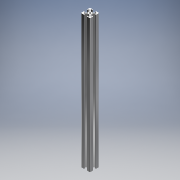
# Autodesk Inventor part: 400mm
Saved by Autodesk Inventor 2017 (Build 210142000, 142)
## iProperties
Part Number: 400mm
Material: Aluminium 6061
Document SubType Name: Modeling
Designer: Till
Density: 2.7 g/cm^3
Appearance: Aluminium - flach
Author: Till
Autodesk Inventor part; units mm, degrees
ref_plane "YZ Plane" through (0, 0, 0) normal (1, 0, 0) x (0, 1, 0)
ref_plane "XZ Plane" through (0, 0, 0) normal (0, 1, 0) x (-1, 0, 0)
ref_plane "XY Plane" through (0, 0, 0) normal (0, 0, 1) x (1, 0, 0)
sketch "Skizze1" plane through (0, 0, 0) normal (0, 0, 1) x (1, 0, 0)
  circle A0 centre (0, 0) radius 2.15
  line L0 (-3.5, -9.5) -> (-3.5, -10)
  line L1 (-3, -9.5) -> (-3.5, -9.5)
  line L2 (-3, -8.3) -> (-3, -9.5)
  line L3 (-5.2994, -8.3) -> (-3, -8.3)
  arc A1 (-5.7944, -7.105) -> (-5.2994, -8.3) centre (-5.2994, -7.6) ccw
  line L4 (-2.1755, -3.4861) -> (-5.7944, -7.105)
  arc A2 (-1.6076, -3.388) -> (-2.1755, -3.4861) centre (-1.8219, -3.8397) ccw
  arc A3 (-1.6076, -3.388) -> (-0.3, -3.738) centre (0, 0) ccw
  line L5 (0, -3.45) -> (-0.3, -3.738)
  line L6 (0.3, -3.738) -> (0, -3.45)
  arc A4 (0.3, -3.738) -> (1.6076, -3.388) centre (0, 0) ccw
  arc A5 (2.1755, -3.4861) -> (1.6076, -3.388) centre (1.8219, -3.8397) ccw
  line L7 (5.7944, -7.105) -> (2.1755, -3.4861)
  arc A6 (5.2994, -8.3) -> (5.7944, -7.105) centre (5.2994, -7.6) ccw
  line L8 (3, -8.3) -> (5.2994, -8.3)
  line L9 (3, -9.5) -> (3, -8.3)
  line L10 (3.5, -9.5) -> (3, -9.5)
  line L11 (3.5, -10) -> (3.5, -9.5)
  line L12 (8.5, -10) -> (3.5, -10)
  arc A7 (8.5, -10) -> (10, -8.5) centre (8.5, -8.5) ccw
  line L13 (10, -3.5) -> (10, -8.5)
  line L14 (9.5, -3.5) -> (10, -3.5)
  line L15 (9.5, -3) -> (9.5, -3.5)
  line L16 (8.3, -3) -> (9.5, -3)
  line L17 (8.3, -5.2994) -> (8.3, -3)
  arc A8 (7.105, -5.7944) -> (8.3, -5.2994) centre (7.6, -5.2994) ccw
  line L18 (3.4861, -2.1755) -> (7.105, -5.7944)
  arc A9 (3.388, -1.6076) -> (3.4861, -2.1755) centre (3.8397, -1.8219) ccw
  arc A10 (3.388, -1.6076) -> (3.738, -0.3) centre (0, 0) ccw
  line L19 (3.45, 0) -> (3.738, -0.3)
  line L20 (3.738, 0.3) -> (3.45, 0)
  arc A11 (3.738, 0.3) -> (3.388, 1.6076) centre (0, 0) ccw
  arc A12 (3.4861, 2.1755) -> (3.388, 1.6076) centre (3.8397, 1.8219) ccw
  line L21 (7.105, 5.7944) -> (3.4861, 2.1755)
  arc A13 (8.3, 5.2994) -> (7.105, 5.7944) centre (7.6, 5.2994) ccw
  line L22 (8.3, 3) -> (8.3, 5.2994)
  line L23 (9.5, 3) -> (8.3, 3)
  line L24 (9.5, 3.5) -> (9.5, 3)
  line L25 (10, 3.5) -> (9.5, 3.5)
  line L26 (10, 8.5) -> (10, 3.5)
  arc A14 (10, 8.5) -> (8.5, 10) centre (8.5, 8.5) ccw
  line L27 (3.5, 10) -> (8.5, 10)
  line L28 (3.5, 9.5) -> (3.5, 10)
  line L29 (3, 9.5) -> (3.5, 9.5)
  line L30 (3, 8.3) -> (3, 9.5)
  line L31 (5.2994, 8.3) -> (3, 8.3)
  arc A15 (5.7944, 7.105) -> (5.2994, 8.3) centre (5.2994, 7.6) ccw
  line L32 (2.1755, 3.4861) -> (5.7944, 7.105)
  arc A16 (1.6076, 3.388) -> (2.1755, 3.4861) centre (1.8219, 3.8397) ccw
  arc A17 (1.6076, 3.388) -> (0.3, 3.738) centre (0, 0) ccw
  line L33 (0, 3.45) -> (0.3, 3.738)
  line L34 (-0.3, 3.738) -> (0, 3.45)
  arc A18 (-0.3, 3.738) -> (-1.6076, 3.388) centre (0, 0) ccw
  arc A19 (-2.1755, 3.4861) -> (-1.6076, 3.388) centre (-1.8219, 3.8397) ccw
  line L35 (-5.7944, 7.105) -> (-2.1755, 3.4861)
  arc A20 (-5.2994, 8.3) -> (-5.7944, 7.105) centre (-5.2994, 7.6) ccw
  line L36 (-3, 8.3) -> (-5.2994, 8.3)
  line L37 (-3, 9.5) -> (-3, 8.3)
  line L38 (-3.5, 9.5) -> (-3, 9.5)
  line L39 (-3.5, 10) -> (-3.5, 9.5)
  line L40 (-8.5, 10) -> (-3.5, 10)
  arc A21 (-8.5, 10) -> (-10, 8.5) centre (-8.5, 8.5) ccw
  line L41 (-10, 3.5) -> (-10, 8.5)
  line L42 (-9.5, 3.5) -> (-10, 3.5)
  line L43 (-9.5, 3) -> (-9.5, 3.5)
  line L44 (-8.3, 3) -> (-9.5, 3)
  line L45 (-8.3, 5.2994) -> (-8.3, 3)
  arc A22 (-7.105, 5.7944) -> (-8.3, 5.2994) centre (-7.6, 5.2994) ccw
  line L46 (-3.4861, 2.1755) -> (-7.105, 5.7944)
  arc A23 (-3.388, 1.6076) -> (-3.4861, 2.1755) centre (-3.8397, 1.8219) ccw
  arc A24 (-3.388, 1.6076) -> (-3.738, 0.3) centre (0, 0) ccw
  line L47 (-3.45, 0) -> (-3.738, 0.3)
  line L48 (-3.738, -0.3) -> (-3.45, 0)
  arc A25 (-3.738, -0.3) -> (-3.388, -1.6076) centre (0, 0) ccw
  arc A26 (-3.4861, -2.1755) -> (-3.388, -1.6076) centre (-3.8397, -1.8219) ccw
  line L49 (-7.105, -5.7944) -> (-3.4861, -2.1755)
  arc A27 (-8.3, -5.2994) -> (-7.105, -5.7944) centre (-7.6, -5.2994) ccw
  line L50 (-8.3, -3) -> (-8.3, -5.2994)
  line L51 (-9.5, -3) -> (-8.3, -3)
  line L52 (-9.5, -3.5) -> (-9.5, -3)
  line L53 (-10, -3.5) -> (-9.5, -3.5)
  line L54 (-10, -8.5) -> (-10, -3.5)
  arc A28 (-10, -8.5) -> (-8.5, -10) centre (-8.5, -8.5) ccw
  line L55 (-3.5, -10) -> (-8.5, -10)
  point P0 (18.4588, -14.4564)
  constraints: 112 end point, 56 point on circle, 29 centre point
extrude "Extrusion1" add sketch "Skizze1" along normal blind 285
